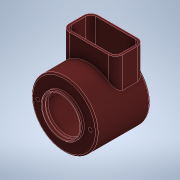
# Autodesk Inventor part: BodyStructure LumbarSupport
Saved by Autodesk Inventor 2022.2 (Build 262287000, 287)
## iProperties
Created: 2022-01-28
Part Number: BodyStructure LumbarSupport
Material: Generic
Document SubType Name: Modeling
Designer: Jochen
Density: 1 g/cm^3
Appearance: Default
Author: Jochen
Autodesk Inventor part; units mm, degrees
ref_plane "YZ Plane" through (0, 0, 0) normal (1, 0, 0) x (0, 1, 0)
ref_plane "XZ Plane" through (0, 0, 0) normal (0, 1, 0) x (-1, 0, 0)
ref_plane "XY Plane" through (0, 0, 0) normal (0, 0, 1) x (1, 0, 0)
sketch "Sketch1" plane through (0, 0, 0) normal (0, 0, 1) x (1, 0, 0)
  line L0 (0, -33.8) -> (0, 45.3) construction
  line L1 (-31.5, 0) -> (31.5, 0) construction
  circle A0 centre (0, 0) radius 13
  line L2 (18.5, 34) -> (-18.5, 34)
  line L3 (-18.5, 34) -> (-18.5, 12.8062)
  line L4 (18.5, 12.8062) -> (18.5, 34)
  circle A1 centre (0, 0) radius 22.5
  circle A2 centre (0, 0) radius 18 construction
  circle A3 centre (-18, 0) radius 1.325
  circle A4 centre (18, 0) radius 1.325
  dimension "d2" = 26
  dimension "d17" = 45
  dimension "d18" = 37
  dimension "d19" = 34
  dimension "d20" = 36
  dimension "d21" = 2.65
  constraints: 6 end point, 5 centre point, 4 point on circle, 2 coincident, 2 point on line, 1 equal radius, 1 horizontal, 1 parallel, 1 perpendicular, 1 other
  measures "d2" diameter of A0
  measures "d17" diameter of A1
  measures "d18" distance of L2.start L2.end
  measures "d19" distance between parallel lines of L1 L2
  measures "d20" diameter of A2
  measures "d21" diameter of A3
extrude "Extrusion1" add sketch "Sketch1" along normal blind 37 contours A0 | A1
extrude "Extrusion2" add sketch "Sketch1" along normal blind 20 separate body contours L4 A1 L3 L2
fillet "Fillet1" radius 5 4 edges at (-18.5, 23.4031, 0) (18.5, 23.4031, 0) (-18.5, 23.4031, 20) (18.5, 23.4031, 20)
combine bodies "Combine1" operation type add bodies to combine 2 1
fillet "Fillet2" radius 1 3 edges at (-22.5, 0, 37) (20.1246, 10.0623, 0) (-10.0623, -20.1246, 0)
sketch "Sketch2" plane through (13.5, 34, 0) normal (0, 0, -1) x (-1, 0, 0)
  circle A0 centre (13.5, -34) radius 14
  circle A1 centre (13.5, -34) radius 13 projected
  dimension "d10" = 28
  constraints: 1 centre point, 1 coincident
  measures "d10" diameter of A0
extrude "Extrusion3" add sketch "Sketch2" along normal blind 0.8 bodies 2
extrude "Extrusion4" add sketch "Sketch2" against normal blind 2 from surface at -37 bodies 2
shell "Shell2" thickness 1.5 removed faces 3 at (-4.5, 34, 13.3333) at (-1.5366, -1.6953, 37) at (-1.5366, -1.6953, 0) bodies 2
chamfer "Chamfer1" distance 0.5 angle 45 2 edges at (14, 0, 39) (14, 0, -0.8)
body "Solid2"
